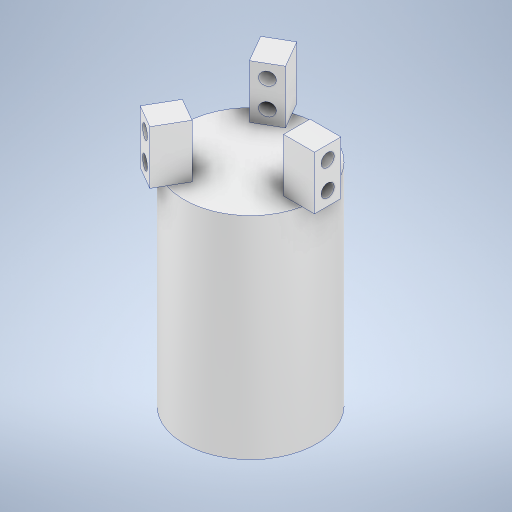
# Autodesk Inventor part: Cilindro
Saved by Autodesk Inventor 2024 (Build 280153000, 153)
## iProperties
Created: 2023-12-04
Part Number: Cilindro
Material: Aluminum 6061
Document SubType Name: Modeling
Designer: Juan_Daleman
Density: 2.7 g/cm^3
Appearance: Aluminum - Flat
Author: Juan_Daleman
Autodesk Inventor part; units mm, degrees
ref_plane "YZ Plane" through (0, 0, 0) normal (1, 0, 0) x (0, 1, 0)
ref_plane "XZ Plane" through (0, 0, 0) normal (0, 1, 0) x (-1, 0, 0)
ref_plane "XY Plane" through (0, 0, 0) normal (0, 0, 1) x (1, 0, 0)
sketch "Sketch1" plane through (0, 0, 0) normal (0, 1, 0) x (-1, 0, 0)
  circle A0 centre (0, 0) radius 15
  dimension "d0" = 30
  constraints: 1 centre point, 1 coincident
  measures "d0" diameter of A0
extrude "Extrusion1" add sketch "Sketch1" along normal blind 47.9
sketch "Sketch2" plane through (0, 47.9, 0) normal (0, 1, 0) x (1, 0, 0)
  circle A0 centre (0, 0) radius 10.5
  line L0 (10.5, 0) -> (10.5, 3)
  line L1 (10.5, 3) -> (17.5, 3)
  line L2 (17.5, 3) -> (17.5, -3)
  line L3 (17.5, -3) -> (10.5, -3)
  line L4 (10.5, -3) -> (10.5, 0)
  line L5 (-5.25, 9.0933) -> (-7.8481, 7.5933)
  line L6 (-7.8481, 7.5933) -> (-11.3481, 13.6554)
  line L7 (-11.3481, 13.6554) -> (-6.1519, 16.6554)
  line L8 (-6.1519, 16.6554) -> (-2.6519, 10.5933)
  line L9 (-2.6519, 10.5933) -> (-5.25, 9.0933)
  line L10 (-5.25, -9.0933) -> (-2.6519, -10.5933)
  line L11 (-2.6519, -10.5933) -> (-6.1519, -16.6554)
  line L12 (-6.1519, -16.6554) -> (-11.3481, -13.6554)
  line L13 (-11.3481, -13.6554) -> (-7.8481, -7.5933)
  line L14 (-7.8481, -7.5933) -> (-5.25, -9.0933)
  line L15 (0, 0) -> (-5.25, 9.0933)
  line L16 (0, 0) -> (10.5, 0)
  dimension "d4" = 21
  dimension "d5" = 3
  dimension "d6" = 7
  dimension "d7" = 6
  dimension "d10" = 360
  dimension "d12" = 120
  constraints: 34 end point, 4 perpendicular, 4 point on line, 2 point on circle, 1 centre point, 1 tangent, 1 vertical, 31 other
  measures "d4" diameter of A0
  measures "d5" distance of L0.start L0.end
  measures "d6" distance of L0.end L1.end
  measures "d7" distance of L1.end L2.end
  measures "d12" angle of L16 L15
extrude "Extrusion2" add sketch "Sketch2" along normal blind 12.1 contours L10 L11 L12 L13 L14 | L5 L6 L7 L8 L9 | L0 L1 L2 L3 L4
sketch "Sketch4" plane through (17.5, 47.9, 3) normal (1, 0, 0) x (0, 0, -1)
  line L0 (6, 12.1) -> (0, 12.1) projected
  line L1 (3, 12.1) -> (3, 9.1)
  line L2 (3, 9.1) -> (3, 3.1)
  circle A0 centre (3, 9.1) radius 1.5
  circle A1 centre (3, 3.1) radius 1.5
  point P0 (3, -47.9)
  dimension "d15" = 3
  dimension "d16" = 6
  dimension "d17" = 3
  dimension "d18" = 3
  constraints: 4 end point, 2 centre point, 2 coincident, 1 midpoint, 1 point on line, 1 vertical
  measures "d15" distance of L1.start L1.end
  measures "d16" distance of L1.end L2.end
  measures "d17" diameter of A0
  measures "d18" diameter of A1
extrude "Extrusion3" cut sketch "Sketch4" against normal through all
sketch "Sketch5" plane through (-6.1519, 47.9, 16.6554) normal (-0.5, 0, 0.866) x (0.866, 0, 0.5)
  line L0 (-6, 12.1) -> (0, 12.1) projected
  line L1 (-3, 12.1) -> (-3, 9.1)
  line L2 (-3, 9.1) -> (-3, 3.1)
  circle A0 centre (-3, 9.1) radius 1.5
  circle A1 centre (-3, 3.1) radius 1.5
  point P0 (-3, -47.9)
  dimension "d21" = 3
  dimension "d22" = 6
  dimension "d23" = 3
  dimension "d24" = 3
  constraints: 4 end point, 2 centre point, 2 coincident, 1 midpoint, 1 point on line, 1 vertical
  measures "d21" distance of L1.start L1.end
  measures "d22" distance of L1.end L2.end
  measures "d23" diameter of A0
  measures "d24" diameter of A1
extrude "Extrusion4" cut sketch "Sketch5" against normal through all
sketch "Sketch6" plane through (-11.3481, 47.9, -13.6554) normal (-0.5, 0, -0.866) x (-0.866, 0, 0.5)
  line L0 (8.2279, 0) -> (-14.2279, 0) projected
  line L1 (0, 12.1) -> (-6, 12.1) projected
  line L2 (-3, 12.1) -> (-3, 9.1)
  line L3 (-3, 9.1) -> (-3, 3.1)
  circle A0 centre (-3, 9.1) radius 1.5
  circle A1 centre (-3, 3.1) radius 1.5
  point P0 (-3, -47.9)
  dimension "d27" = 3
  dimension "d28" = 6
  dimension "d29" = 3
  dimension "d30" = 3
  constraints: 4 end point, 2 centre point, 2 coincident, 1 midpoint, 1 point on line, 1 vertical
  measures "d27" distance of L2.start L2.end
  measures "d28" distance of L2.end L3.end
  measures "d29" diameter of A0
  measures "d30" diameter of A1
extrude "Extrusion5" cut sketch "Sketch6" against normal through all
body "Solid1"
